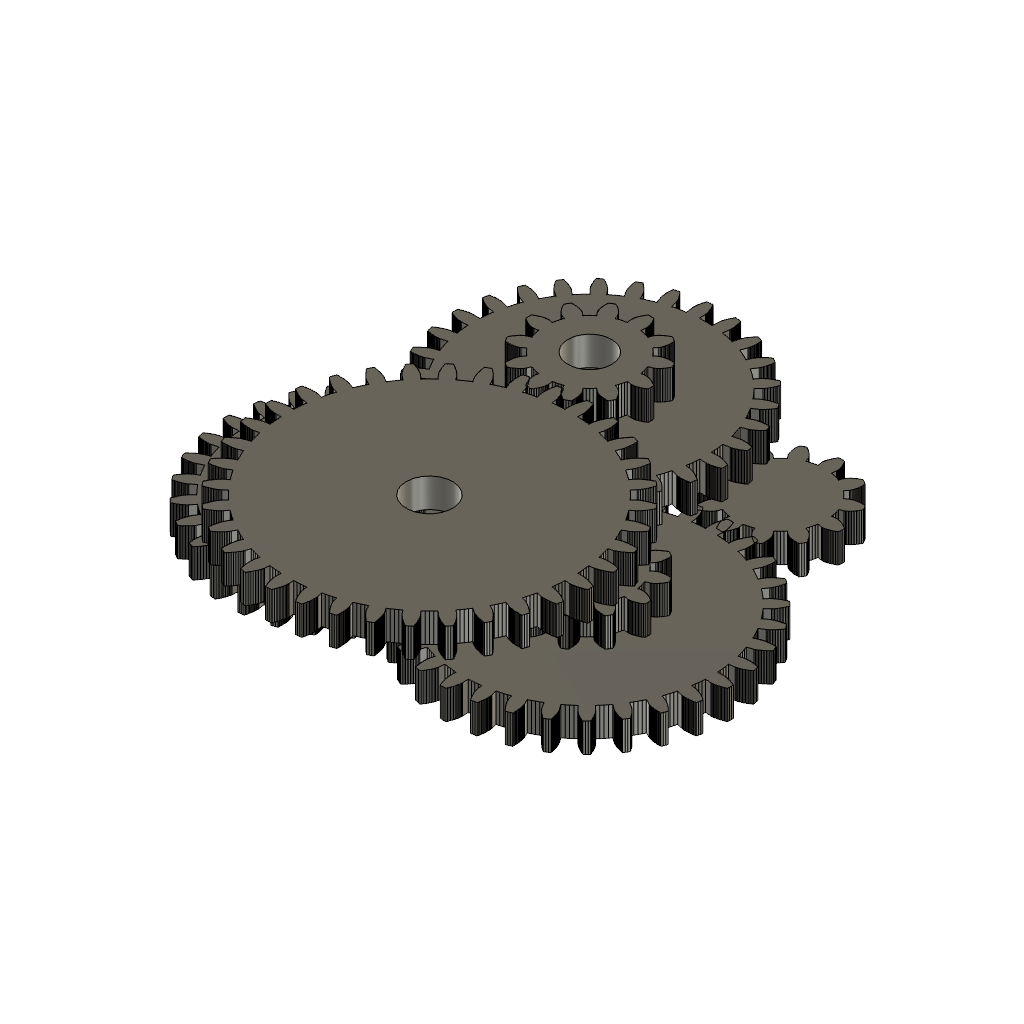
Infidex176V-IDENTIDEM.design-remix-counter-train (Autodesk Fusion 360 design; units mm, degrees)
part number: 2026-09-16-11-02-38-314
part number: 2026-09-16-11-02-48-603
part number: 2026-09-16-11-02-48-989
part number: 2026-09-16-11-02-51-230
part number: 2026-09-16-11-02-54-507
part number: 2026-09-16-11-02-59-213
Autodesk Fusion 360 part; units mm, degrees
(part 1 of 7)
ref_plane "WorkPlane1" through (0, 0, 36.8) normal (0, 0, 1) x (1, 0, 0) in component "CT sprocket pinion (tool body)"
sketch "Sketch1" plane through (0, 0, 36.8) normal (0, 0, 1) x (1, 0, 0) in component "CT sprocket pinion (tool body)"
  line L0 (76.254, -45.68) -> (76.5435, -45.7246)
  line L1 (76.5435, -45.7246) -> (76.6148, -45.7257)
  line L2 (76.6148, -45.7257) -> (76.6872, -45.7186)
  line L3 (76.6872, -45.7186) -> (76.7603, -45.7057)
  line L4 (76.7603, -45.7057) -> (76.834, -45.688)
  line L5 (76.834, -45.688) -> (76.9079, -45.6659)
  line L6 (76.9079, -45.6659) -> (76.9821, -45.6396)
  line L7 (76.9821, -45.6396) -> (77.0564, -45.6095)
  line L8 (77.0564, -45.6095) -> (77.1307, -45.5756)
  line L9 (77.1307, -45.5756) -> (77.2048, -45.538)
  line L10 (77.2048, -45.538) -> (77.2787, -45.4969)
  line L11 (77.2787, -45.4969) -> (77.3523, -45.4524)
  line L12 (77.3523, -45.4524) -> (77.4255, -45.4044)
  line L13 (77.4255, -45.4044) -> (77.4295, -45.2748)
  line L14 (77.4295, -45.2748) -> (77.4295, -45.1452)
  line L15 (77.4295, -45.1452) -> (77.4255, -45.0156)
  line L16 (77.4255, -45.0156) -> (77.3523, -44.9676)
  line L17 (77.3523, -44.9676) -> (77.2787, -44.9231)
  line L18 (77.2787, -44.9231) -> (77.2048, -44.882)
  line L19 (77.2048, -44.882) -> (77.1307, -44.8444)
  line L20 (77.1307, -44.8444) -> (77.0564, -44.8105)
  line L21 (77.0564, -44.8105) -> (76.9821, -44.7804)
  line L22 (76.9821, -44.7804) -> (76.9079, -44.7541)
  line L23 (76.9079, -44.7541) -> (76.834, -44.732)
  line L24 (76.834, -44.732) -> (76.7603, -44.7143)
  line L25 (76.7603, -44.7143) -> (76.6872, -44.7014)
  line L26 (76.6872, -44.7014) -> (76.6148, -44.6943)
  line L27 (76.6148, -44.6943) -> (76.5435, -44.6954)
  line L28 (76.5435, -44.6954) -> (76.254, -44.74)
  line L29 (76.254, -44.74) -> (76.2239, -44.5742)
  line L30 (76.2239, -44.5742) -> (76.1847, -44.4102)
  line L31 (76.1847, -44.4102) -> (76.1367, -44.2487)
  line L32 (76.1367, -44.2487) -> (76.0799, -44.09)
  line L33 (76.0799, -44.09) -> (76.3529, -43.9839)
  line L34 (76.3529, -43.9839) -> (76.4151, -43.9492)
  line L35 (76.4151, -43.9492) -> (76.4743, -43.9068)
  line L36 (76.4743, -43.9068) -> (76.5312, -43.8591)
  line L37 (76.5312, -43.8591) -> (76.5861, -43.807)
  line L38 (76.5861, -43.807) -> (76.6391, -43.7508)
  line L39 (76.6391, -43.7508) -> (76.6902, -43.691)
  line L40 (76.6902, -43.691) -> (76.7395, -43.6278)
  line L41 (76.7395, -43.6278) -> (76.7868, -43.5613)
  line L42 (76.7868, -43.5613) -> (76.8323, -43.4917)
  line L43 (76.8323, -43.4917) -> (76.8758, -43.4191)
  line L44 (76.8758, -43.4191) -> (76.9172, -43.3437)
  line L45 (76.9172, -43.3437) -> (76.9566, -43.2656)
  line L46 (76.9566, -43.2656) -> (76.8953, -43.1514)
  line L47 (76.8953, -43.1514) -> (76.8305, -43.0391)
  line L48 (76.8305, -43.0391) -> (76.7622, -42.9289)
  line L49 (76.7622, -42.9289) -> (76.6749, -42.9239)
  line L50 (76.6749, -42.9239) -> (76.5888, -42.9221)
  line L51 (76.5888, -42.9221) -> (76.5042, -42.9235)
  line L52 (76.5042, -42.9235) -> (76.4213, -42.9281)
  line L53 (76.4213, -42.9281) -> (76.34, -42.9358)
  line L54 (76.34, -42.9358) -> (76.2606, -42.9469)
  line L55 (76.2606, -42.9469) -> (76.1832, -42.9612)
  line L56 (76.1832, -42.9612) -> (76.1081, -42.9791)
  line L57 (76.1081, -42.9791) -> (76.0355, -43.0005)
  line L58 (76.0355, -43.0005) -> (75.9657, -43.026)
  line L59 (75.9657, -43.026) -> (75.8994, -43.056)
  line L60 (75.8994, -43.056) -> (75.8383, -43.0926)
  line L61 (75.8383, -43.0926) -> (75.6099, -43.2759)
  line L62 (75.6099, -43.2759) -> (75.5008, -43.1474)
  line L63 (75.5008, -43.1474) -> (75.385, -43.025)
  line L64 (75.385, -43.025) -> (75.2626, -42.9092)
  line L65 (75.2626, -42.9092) -> (75.1341, -42.8001)
  line L66 (75.1341, -42.8001) -> (75.3174, -42.5717)
  line L67 (75.3174, -42.5717) -> (75.354, -42.5106)
  line L68 (75.354, -42.5106) -> (75.384, -42.4443)
  line L69 (75.384, -42.4443) -> (75.4095, -42.3745)
  line L70 (75.4095, -42.3745) -> (75.4309, -42.3019)
  line L71 (75.4309, -42.3019) -> (75.4488, -42.2268)
  line L72 (75.4488, -42.2268) -> (75.4631, -42.1494)
  line L73 (75.4631, -42.1494) -> (75.4742, -42.07)
  line L74 (75.4742, -42.07) -> (75.4819, -41.9887)
  line L75 (75.4819, -41.9887) -> (75.4865, -41.9058)
  line L76 (75.4865, -41.9058) -> (75.4879, -41.8212)
  line L77 (75.4879, -41.8212) -> (75.4861, -41.7351)
  line L78 (75.4861, -41.7351) -> (75.4811, -41.6478)
  line L79 (75.4811, -41.6478) -> (75.3709, -41.5795)
  line L80 (75.3709, -41.5795) -> (75.2586, -41.5147)
  line L81 (75.2586, -41.5147) -> (75.1444, -41.4534)
  line L82 (75.1444, -41.4534) -> (75.0663, -41.4928)
  line L83 (75.0663, -41.4928) -> (74.9909, -41.5342)
  line L84 (74.9909, -41.5342) -> (74.9183, -41.5777)
  line L85 (74.9183, -41.5777) -> (74.8487, -41.6232)
  line L86 (74.8487, -41.6232) -> (74.7822, -41.6705)
  line L87 (74.7822, -41.6705) -> (74.719, -41.7198)
  line L88 (74.719, -41.7198) -> (74.6592, -41.7709)
  line L89 (74.6592, -41.7709) -> (74.603, -41.8239)
  line L90 (74.603, -41.8239) -> (74.5509, -41.8788)
  line L91 (74.5509, -41.8788) -> (74.5032, -41.9357)
  line L92 (74.5032, -41.9357) -> (74.4608, -41.9949)
  line L93 (74.4608, -41.9949) -> (74.4261, -42.0571)
  line L94 (74.4261, -42.0571) -> (74.32, -42.3301)
  line L95 (74.32, -42.3301) -> (74.1613, -42.2733)
  line L96 (74.1613, -42.2733) -> (73.9998, -42.2253)
  line L97 (73.9998, -42.2253) -> (73.8358, -42.1861)
  line L98 (73.8358, -42.1861) -> (73.67, -42.156)
  line L99 (73.67, -42.156) -> (73.7146, -41.8665)
  line L100 (73.7146, -41.8665) -> (73.7157, -41.7952)
  line L101 (73.7157, -41.7952) -> (73.7086, -41.7228)
  line L102 (73.7086, -41.7228) -> (73.6957, -41.6497)
  line L103 (73.6957, -41.6497) -> (73.678, -41.576)
  line L104 (73.678, -41.576) -> (73.6559, -41.5021)
  line L105 (73.6559, -41.5021) -> (73.6296, -41.4279)
  line L106 (73.6296, -41.4279) -> (73.5995, -41.3536)
  line L107 (73.5995, -41.3536) -> (73.5656, -41.2793)
  line L108 (73.5656, -41.2793) -> (73.528, -41.2052)
  line L109 (73.528, -41.2052) -> (73.4869, -41.1313)
  line L110 (73.4869, -41.1313) -> (73.4424, -41.0577)
  line L111 (73.4424, -41.0577) -> (73.3944, -40.9845)
  line L112 (73.3944, -40.9845) -> (73.2648, -40.9805)
  line L113 (73.2648, -40.9805) -> (73.1352, -40.9805)
  line L114 (73.1352, -40.9805) -> (73.0056, -40.9845)
  line L115 (73.0056, -40.9845) -> (72.9576, -41.0577)
  line L116 (72.9576, -41.0577) -> (72.9131, -41.1313)
  line L117 (72.9131, -41.1313) -> (72.872, -41.2052)
  line L118 (72.872, -41.2052) -> (72.8344, -41.2793)
  line L119 (72.8344, -41.2793) -> (72.8005, -41.3536)
  line L120 (72.8005, -41.3536) -> (72.7704, -41.4279)
  line L121 (72.7704, -41.4279) -> (72.7441, -41.5021)
  line L122 (72.7441, -41.5021) -> (72.722, -41.576)
  line L123 (72.722, -41.576) -> (72.7043, -41.6497)
  line L124 (72.7043, -41.6497) -> (72.6914, -41.7228)
  line L125 (72.6914, -41.7228) -> (72.6843, -41.7952)
  line L126 (72.6843, -41.7952) -> (72.6854, -41.8665)
  line L127 (72.6854, -41.8665) -> (72.73, -42.156)
  line L128 (72.73, -42.156) -> (72.5642, -42.1861)
  line L129 (72.5642, -42.1861) -> (72.4002, -42.2253)
  line L130 (72.4002, -42.2253) -> (72.2387, -42.2733)
  line L131 (72.2387, -42.2733) -> (72.08, -42.3301)
  line L132 (72.08, -42.3301) -> (71.9739, -42.0571)
  line L133 (71.9739, -42.0571) -> (71.9392, -41.9949)
  line L134 (71.9392, -41.9949) -> (71.8968, -41.9357)
  line L135 (71.8968, -41.9357) -> (71.8491, -41.8788)
  line L136 (71.8491, -41.8788) -> (71.797, -41.8239)
  line L137 (71.797, -41.8239) -> (71.7408, -41.7709)
  line L138 (71.7408, -41.7709) -> (71.681, -41.7198)
  line L139 (71.681, -41.7198) -> (71.6178, -41.6705)
  line L140 (71.6178, -41.6705) -> (71.5513, -41.6232)
  line L141 (71.5513, -41.6232) -> (71.4817, -41.5777)
  line L142 (71.4817, -41.5777) -> (71.4091, -41.5342)
  line L143 (71.4091, -41.5342) -> (71.3337, -41.4928)
  line L144 (71.3337, -41.4928) -> (71.2556, -41.4534)
  line L145 (71.2556, -41.4534) -> (71.1414, -41.5147)
  line L146 (71.1414, -41.5147) -> (71.0291, -41.5795)
  line L147 (71.0291, -41.5795) -> (70.9189, -41.6478)
  line L148 (70.9189, -41.6478) -> (70.9139, -41.7351)
  line L149 (70.9139, -41.7351) -> (70.9121, -41.8212)
  line L150 (70.9121, -41.8212) -> (70.9135, -41.9058)
  line L151 (70.9135, -41.9058) -> (70.9181, -41.9887)
  line L152 (70.9181, -41.9887) -> (70.9258, -42.07)
  line L153 (70.9258, -42.07) -> (70.9369, -42.1494)
  line L154 (70.9369, -42.1494) -> (70.9512, -42.2268)
  line L155 (70.9512, -42.2268) -> (70.9691, -42.3019)
  line L156 (70.9691, -42.3019) -> (70.9905, -42.3745)
  line L157 (70.9905, -42.3745) -> (71.016, -42.4443)
  line L158 (71.016, -42.4443) -> (71.046, -42.5106)
  line L159 (71.046, -42.5106) -> (71.0826, -42.5717)
  line L160 (71.0826, -42.5717) -> (71.2659, -42.8001)
  line L161 (71.2659, -42.8001) -> (71.1374, -42.9092)
  line L162 (71.1374, -42.9092) -> (71.015, -43.025)
  line L163 (71.015, -43.025) -> (70.8992, -43.1474)
  line L164 (70.8992, -43.1474) -> (70.7901, -43.2759)
  line L165 (70.7901, -43.2759) -> (70.5617, -43.0926)
  line L166 (70.5617, -43.0926) -> (70.5006, -43.056)
  line L167 (70.5006, -43.056) -> (70.4343, -43.026)
  line L168 (70.4343, -43.026) -> (70.3645, -43.0005)
  line L169 (70.3645, -43.0005) -> (70.2919, -42.9791)
  line L170 (70.2919, -42.9791) -> (70.2168, -42.9612)
  line L171 (70.2168, -42.9612) -> (70.1394, -42.9469)
  line L172 (70.1394, -42.9469) -> (70.06, -42.9358)
  line L173 (70.06, -42.9358) -> (69.9787, -42.9281)
  line L174 (69.9787, -42.9281) -> (69.8958, -42.9235)
  line L175 (69.8958, -42.9235) -> (69.8112, -42.9221)
  line L176 (69.8112, -42.9221) -> (69.7251, -42.9239)
  line L177 (69.7251, -42.9239) -> (69.6378, -42.9289)
  line L178 (69.6378, -42.9289) -> (69.5695, -43.0391)
  line L179 (69.5695, -43.0391) -> (69.5047, -43.1514)
  line L180 (69.5047, -43.1514) -> (69.4434, -43.2656)
  line L181 (69.4434, -43.2656) -> (69.4828, -43.3437)
  line L182 (69.4828, -43.3437) -> (69.5242, -43.4191)
  line L183 (69.5242, -43.4191) -> (69.5677, -43.4917)
  line L184 (69.5677, -43.4917) -> (69.6132, -43.5613)
  line L185 (69.6132, -43.5613) -> (69.6605, -43.6278)
  line L186 (69.6605, -43.6278) -> (69.7098, -43.691)
  line L187 (69.7098, -43.691) -> (69.7609, -43.7508)
  line L188 (69.7609, -43.7508) -> (69.8139, -43.807)
  line L189 (69.8139, -43.807) -> (69.8688, -43.8591)
  line L190 (69.8688, -43.8591) -> (69.9257, -43.9068)
  line L191 (69.9257, -43.9068) -> (69.9849, -43.9492)
  line L192 (69.9849, -43.9492) -> (70.0471, -43.9839)
  line L193 (70.0471, -43.9839) -> (70.3201, -44.09)
  line L194 (70.3201, -44.09) -> (70.2633, -44.2487)
  line L195 (70.2633, -44.2487) -> (70.2153, -44.4102)
  line L196 (70.2153, -44.4102) -> (70.1761, -44.5742)
  line L197 (70.1761, -44.5742) -> (70.146, -44.74)
  line L198 (70.146, -44.74) -> (69.8565, -44.6954)
  line L199 (69.8565, -44.6954) -> (69.7852, -44.6943)
  line L200 (69.7852, -44.6943) -> (69.7128, -44.7014)
  line L201 (69.7128, -44.7014) -> (69.6397, -44.7143)
  line L202 (69.6397, -44.7143) -> (69.566, -44.732)
  line L203 (69.566, -44.732) -> (69.4921, -44.7541)
  line L204 (69.4921, -44.7541) -> (69.4179, -44.7804)
  line L205 (69.4179, -44.7804) -> (69.3436, -44.8105)
  line L206 (69.3436, -44.8105) -> (69.2693, -44.8444)
  line L207 (69.2693, -44.8444) -> (69.1952, -44.882)
  line L208 (69.1952, -44.882) -> (69.1213, -44.9231)
  line L209 (69.1213, -44.9231) -> (69.0477, -44.9676)
  line L210 (69.0477, -44.9676) -> (68.9745, -45.0156)
  line L211 (68.9745, -45.0156) -> (68.9705, -45.1452)
  line L212 (68.9705, -45.1452) -> (68.9705, -45.2748)
  line L213 (68.9705, -45.2748) -> (68.9745, -45.4044)
  line L214 (68.9745, -45.4044) -> (69.0477, -45.4524)
  line L215 (69.0477, -45.4524) -> (69.1213, -45.4969)
  line L216 (69.1213, -45.4969) -> (69.1952, -45.538)
  line L217 (69.1952, -45.538) -> (69.2693, -45.5756)
  line L218 (69.2693, -45.5756) -> (69.3436, -45.6095)
  line L219 (69.3436, -45.6095) -> (69.4179, -45.6396)
  line L220 (69.4179, -45.6396) -> (69.4921, -45.6659)
  line L221 (69.4921, -45.6659) -> (69.566, -45.688)
  line L222 (69.566, -45.688) -> (69.6397, -45.7057)
  line L223 (69.6397, -45.7057) -> (69.7128, -45.7186)
  line L224 (69.7128, -45.7186) -> (69.7852, -45.7257)
  line L225 (69.7852, -45.7257) -> (69.8565, -45.7246)
  line L226 (69.8565, -45.7246) -> (70.146, -45.68)
  line L227 (70.146, -45.68) -> (70.1761, -45.8458)
  line L228 (70.1761, -45.8458) -> (70.2153, -46.0098)
  line L229 (70.2153, -46.0098) -> (70.2633, -46.1713)
  line L230 (70.2633, -46.1713) -> (70.3201, -46.33)
  line L231 (70.3201, -46.33) -> (70.0471, -46.4361)
  line L232 (70.0471, -46.4361) -> (69.9849, -46.4708)
  line L233 (69.9849, -46.4708) -> (69.9257, -46.5132)
  line L234 (69.9257, -46.5132) -> (69.8688, -46.5609)
  line L235 (69.8688, -46.5609) -> (69.8139, -46.613)
  line L236 (69.8139, -46.613) -> (69.7609, -46.6692)
  line L237 (69.7609, -46.6692) -> (69.7098, -46.729)
  line L238 (69.7098, -46.729) -> (69.6605, -46.7922)
  line L239 (69.6605, -46.7922) -> (69.6132, -46.8587)
  line L240 (69.6132, -46.8587) -> (69.5677, -46.9283)
  line L241 (69.5677, -46.9283) -> (69.5242, -47.0009)
  line L242 (69.5242, -47.0009) -> (69.4828, -47.0763)
  line L243 (69.4828, -47.0763) -> (69.4434, -47.1544)
  line L244 (69.4434, -47.1544) -> (69.5047, -47.2686)
  line L245 (69.5047, -47.2686) -> (69.5695, -47.3809)
  line L246 (69.5695, -47.3809) -> (69.6378, -47.4911)
  line L247 (69.6378, -47.4911) -> (69.7251, -47.4961)
  line L248 (69.7251, -47.4961) -> (69.8112, -47.4979)
  line L249 (69.8112, -47.4979) -> (69.8958, -47.4965)
  line L250 (69.8958, -47.4965) -> (69.9787, -47.4919)
  line L251 (69.9787, -47.4919) -> (70.06, -47.4842)
  line L252 (70.06, -47.4842) -> (70.1394, -47.4731)
  line L253 (70.1394, -47.4731) -> (70.2168, -47.4588)
  line L254 (70.2168, -47.4588) -> (70.2919, -47.4409)
  line L255 (70.2919, -47.4409) -> (70.3645, -47.4195)
  line L256 (70.3645, -47.4195) -> (70.4343, -47.394)
  line L257 (70.4343, -47.394) -> (70.5006, -47.364)
  line L258 (70.5006, -47.364) -> (70.5617, -47.3274)
  line L259 (70.5617, -47.3274) -> (70.7901, -47.1441)
  line L260 (70.7901, -47.1441) -> (70.8992, -47.2726)
  line L261 (70.8992, -47.2726) -> (71.015, -47.395)
  line L262 (71.015, -47.395) -> (71.1374, -47.5108)
  line L263 (71.1374, -47.5108) -> (71.2659, -47.6199)
  line L264 (71.2659, -47.6199) -> (71.0826, -47.8483)
  line L265 (71.0826, -47.8483) -> (71.046, -47.9094)
  line L266 (71.046, -47.9094) -> (71.016, -47.9757)
  line L267 (71.016, -47.9757) -> (70.9905, -48.0455)
  line L268 (70.9905, -48.0455) -> (70.9691, -48.1181)
  line L269 (70.9691, -48.1181) -> (70.9512, -48.1932)
  line L270 (70.9512, -48.1932) -> (70.9369, -48.2706)
  line L271 (70.9369, -48.2706) -> (70.9258, -48.35)
  line L272 (70.9258, -48.35) -> (70.9181, -48.4313)
  line L273 (70.9181, -48.4313) -> (70.9135, -48.5142)
  line L274 (70.9135, -48.5142) -> (70.9121, -48.5988)
  line L275 (70.9121, -48.5988) -> (70.9139, -48.6849)
  line L276 (70.9139, -48.6849) -> (70.9189, -48.7722)
  line L277 (70.9189, -48.7722) -> (71.0291, -48.8405)
  line L278 (71.0291, -48.8405) -> (71.1414, -48.9053)
  line L279 (71.1414, -48.9053) -> (71.2556, -48.9666)
  line L280 (71.2556, -48.9666) -> (71.3337, -48.9272)
  line L281 (71.3337, -48.9272) -> (71.4091, -48.8858)
  line L282 (71.4091, -48.8858) -> (71.4817, -48.8423)
  line L283 (71.4817, -48.8423) -> (71.5513, -48.7968)
  line L284 (71.5513, -48.7968) -> (71.6178, -48.7495)
  line L285 (71.6178, -48.7495) -> (71.681, -48.7002)
  line L286 (71.681, -48.7002) -> (71.7408, -48.6491)
  line L287 (71.7408, -48.6491) -> (71.797, -48.5961)
  line L288 (71.797, -48.5961) -> (71.8491, -48.5412)
  line L289 (71.8491, -48.5412) -> (71.8968, -48.4843)
  line L290 (71.8968, -48.4843) -> (71.9392, -48.4251)
  line L291 (71.9392, -48.4251) -> (71.9739, -48.3629)
  line L292 (71.9739, -48.3629) -> (72.08, -48.0899)
  line L293 (72.08, -48.0899) -> (72.2387, -48.1467)
  line L294 (72.2387, -48.1467) -> (72.4002, -48.1947)
  line L295 (72.4002, -48.1947) -> (72.5642, -48.2339)
  line L296 (72.5642, -48.2339) -> (72.73, -48.264)
  line L297 (72.73, -48.264) -> (72.6854, -48.5535)
  line L298 (72.6854, -48.5535) -> (72.6843, -48.6248)
  line L299 (72.6843, -48.6248) -> (72.6914, -48.6972)
  line L300 (72.6914, -48.6972) -> (72.7043, -48.7703)
  line L301 (72.7043, -48.7703) -> (72.722, -48.844)
  line L302 (72.722, -48.844) -> (72.7441, -48.9179)
  line L303 (72.7441, -48.9179) -> (72.7704, -48.9921)
  line L304 (72.7704, -48.9921) -> (72.8005, -49.0664)
  line L305 (72.8005, -49.0664) -> (72.8344, -49.1407)
  line L306 (72.8344, -49.1407) -> (72.872, -49.2148)
  line L307 (72.872, -49.2148) -> (72.9131, -49.2887)
  line L308 (72.9131, -49.2887) -> (72.9576, -49.3623)
  line L309 (72.9576, -49.3623) -> (73.0056, -49.4355)
  line L310 (73.0056, -49.4355) -> (73.1352, -49.4395)
  line L311 (73.1352, -49.4395) -> (73.2648, -49.4395)
  line L312 (73.2648, -49.4395) -> (73.3944, -49.4355)
  line L313 (73.3944, -49.4355) -> (73.4424, -49.3623)
  line L314 (73.4424, -49.3623) -> (73.4869, -49.2887)
  line L315 (73.4869, -49.2887) -> (73.528, -49.2148)
  line L316 (73.528, -49.2148) -> (73.5656, -49.1407)
  line L317 (73.5656, -49.1407) -> (73.5995, -49.0664)
  line L318 (73.5995, -49.0664) -> (73.6296, -48.9921)
  line L319 (73.6296, -48.9921) -> (73.6559, -48.9179)
  line L320 (73.6559, -48.9179) -> (73.678, -48.844)
  line L321 (73.678, -48.844) -> (73.6957, -48.7703)
  line L322 (73.6957, -48.7703) -> (73.7086, -48.6972)
  line L323 (73.7086, -48.6972) -> (73.7157, -48.6248)
  line L324 (73.7157, -48.6248) -> (73.7146, -48.5535)
  line L325 (73.7146, -48.5535) -> (73.67, -48.264)
  line L326 (73.67, -48.264) -> (73.8358, -48.2339)
  line L327 (73.8358, -48.2339) -> (73.9998, -48.1947)
  line L328 (73.9998, -48.1947) -> (74.1613, -48.1467)
  line L329 (74.1613, -48.1467) -> (74.32, -48.0899)
  line L330 (74.32, -48.0899) -> (74.4261, -48.3629)
  line L331 (74.4261, -48.3629) -> (74.4608, -48.4251)
  line L332 (74.4608, -48.4251) -> (74.5032, -48.4843)
  line L333 (74.5032, -48.4843) -> (74.5509, -48.5412)
  line L334 (74.5509, -48.5412) -> (74.603, -48.5961)
  line L335 (74.603, -48.5961) -> (74.6592, -48.6491)
  line L336 (74.6592, -48.6491) -> (74.719, -48.7002)
  line L337 (74.719, -48.7002) -> (74.7822, -48.7495)
  line L338 (74.7822, -48.7495) -> (74.8487, -48.7968)
  line L339 (74.8487, -48.7968) -> (74.9183, -48.8423)
  line L340 (74.9183, -48.8423) -> (74.9909, -48.8858)
  line L341 (74.9909, -48.8858) -> (75.0663, -48.9272)
  line L342 (75.0663, -48.9272) -> (75.1444, -48.9666)
  line L343 (75.1444, -48.9666) -> (75.2586, -48.9053)
  line L344 (75.2586, -48.9053) -> (75.3709, -48.8405)
  line L345 (75.3709, -48.8405) -> (75.4811, -48.7722)
  line L346 (75.4811, -48.7722) -> (75.4861, -48.6849)
  line L347 (75.4861, -48.6849) -> (75.4879, -48.5988)
  line L348 (75.4879, -48.5988) -> (75.4865, -48.5142)
  line L349 (75.4865, -48.5142) -> (75.4819, -48.4313)
  line L350 (75.4819, -48.4313) -> (75.4742, -48.35)
  line L351 (75.4742, -48.35) -> (75.4631, -48.2706)
  line L352 (75.4631, -48.2706) -> (75.4488, -48.1932)
  line L353 (75.4488, -48.1932) -> (75.4309, -48.1181)
  line L354 (75.4309, -48.1181) -> (75.4095, -48.0455)
  line L355 (75.4095, -48.0455) -> (75.384, -47.9757)
  line L356 (75.384, -47.9757) -> (75.354, -47.9094)
  line L357 (75.354, -47.9094) -> (75.3174, -47.8483)
  line L358 (75.3174, -47.8483) -> (75.1341, -47.6199)
  line L359 (75.1341, -47.6199) -> (75.2626, -47.5108)
  line L360 (75.2626, -47.5108) -> (75.385, -47.395)
  line L361 (75.385, -47.395) -> (75.5008, -47.2726)
  line L362 (75.5008, -47.2726) -> (75.6099, -47.1441)
  line L363 (75.6099, -47.1441) -> (75.8383, -47.3274)
  line L364 (75.8383, -47.3274) -> (75.8994, -47.364)
  line L365 (75.8994, -47.364) -> (75.9657, -47.394)
  line L366 (75.9657, -47.394) -> (76.0355, -47.4195)
  line L367 (76.0355, -47.4195) -> (76.1081, -47.4409)
  line L368 (76.1081, -47.4409) -> (76.1832, -47.4588)
  line L369 (76.1832, -47.4588) -> (76.2606, -47.4731)
  line L370 (76.2606, -47.4731) -> (76.34, -47.4842)
  line L371 (76.34, -47.4842) -> (76.4213, -47.4919)
  line L372 (76.4213, -47.4919) -> (76.5042, -47.4965)
  line L373 (76.5042, -47.4965) -> (76.5888, -47.4979)
  line L374 (76.5888, -47.4979) -> (76.6749, -47.4961)
  line L375 (76.6749, -47.4961) -> (76.7622, -47.4911)
  line L376 (76.7622, -47.4911) -> (76.8305, -47.3809)
  line L377 (76.8305, -47.3809) -> (76.8953, -47.2686)
  line L378 (76.8953, -47.2686) -> (76.9566, -47.1544)
  line L379 (76.9566, -47.1544) -> (76.9172, -47.0763)
  line L380 (76.9172, -47.0763) -> (76.8758, -47.0009)
  line L381 (76.8758, -47.0009) -> (76.8323, -46.9283)
  line L382 (76.8323, -46.9283) -> (76.7868, -46.8587)
  line L383 (76.7868, -46.8587) -> (76.7395, -46.7922)
  line L384 (76.7395, -46.7922) -> (76.6902, -46.729)
  line L385 (76.6902, -46.729) -> (76.6391, -46.6692)
  line L386 (76.6391, -46.6692) -> (76.5861, -46.613)
  line L387 (76.5861, -46.613) -> (76.5312, -46.5609)
  line L388 (76.5312, -46.5609) -> (76.4743, -46.5132)
  line L389 (76.4743, -46.5132) -> (76.4151, -46.4708)
  line L390 (76.4151, -46.4708) -> (76.3529, -46.4361)
  line L391 (76.3529, -46.4361) -> (76.0799, -46.33)
  line L392 (76.0799, -46.33) -> (76.1367, -46.1713)
  line L393 (76.1367, -46.1713) -> (76.1847, -46.0098)
  line L394 (76.1847, -46.0098) -> (76.2239, -45.8458)
  line L395 (76.2239, -45.8458) -> (76.254, -45.68)
extrude "Extrude1" add sketch "Sketch1" along normal blind 2 makes body 1 in component "CT sprocket pinion (tool body)"
ref_plane "WorkPlane1" through (0, 0, 36.8) normal (0, 0, 1) x (1, 0, 0) in component "CT idler 1"
sketch "Sketch1 (2)" plane through (0, 0, 36.8) normal (0, 0, 1) x (1, 0, 0) in component "CT idler 1"
  line L0 (81.6294, -58.8253) -> (82.04, -58.8452)
  line L1 (82.04, -58.8452) -> (82.1151, -58.8424)
  line L2 (82.1151, -58.8424) -> (82.1905, -58.8341)
  line L3 (82.1905, -58.8341) -> (82.2661, -58.8222)
  line L4 (82.2661, -58.8222) -> (82.3417, -58.8073)
  line L5 (82.3417, -58.8073) -> (82.4174, -58.7898)
  line L6 (82.4174, -58.7898) -> (82.4932, -58.7699)
  line L7 (82.4932, -58.7699) -> (82.5689, -58.7477)
  line L8 (82.5689, -58.7477) -> (82.6447, -58.7234)
  line L9 (82.6447, -58.7234) -> (82.7205, -58.6971)
  line L10 (82.7205, -58.6971) -> (82.7962, -58.6689)
  line L11 (82.7962, -58.6689) -> (82.8719, -58.6389)
  line L12 (82.8719, -58.6389) -> (82.9475, -58.607)
  line L13 (82.9475, -58.607) -> (82.9493, -58.4749)
  line L14 (82.9493, -58.4749) -> (82.9493, -58.3429)
  line L15 (82.9493, -58.3429) -> (82.9475, -58.2108)
  line L16 (82.9475, -58.2108) -> (82.8719, -58.1789)
  line L17 (82.8719, -58.1789) -> (82.7962, -58.1489)
  line L18 (82.7962, -58.1489) -> (82.7205, -58.1207)
  line L19 (82.7205, -58.1207) -> (82.6447, -58.0944)
  line L20 (82.6447, -58.0944) -> (82.5689, -58.0701)
  line L21 (82.5689, -58.0701) -> (82.4932, -58.0479)
  line L22 (82.4932, -58.0479) -> (82.4174, -58.028)
  line L23 (82.4174, -58.028) -> (82.3417, -58.0105)
  line L24 (82.3417, -58.0105) -> (82.2661, -57.9956)
  line L25 (82.2661, -57.9956) -> (82.1905, -57.9837)
  line L26 (82.1905, -57.9837) -> (82.1151, -57.9754)
  line L27 (82.1151, -57.9754) -> (82.04, -57.9726)
  line L28 (82.04, -57.9726) -> (81.6294, -57.9925)
  line L29 (81.6294, -57.9925) -> (81.6164, -57.7785)
  line L30 (81.6164, -57.7785) -> (81.5981, -57.565)
  line L31 (81.5981, -57.565) -> (81.5744, -57.3519)
  line L32 (81.5744, -57.3519) -> (81.5454, -57.1395)
  line L33 (81.5454, -57.1395) -> (81.952, -57.0789)
  line L34 (81.952, -57.0789) -> (82.0251, -57.0615)
  line L35 (82.0251, -57.0615) -> (82.0975, -57.0387)
  line L36 (82.0975, -57.0387) -> (82.1692, -57.0123)
  line L37 (82.1692, -57.0123) -> (82.2405, -56.9829)
  line L38 (82.2405, -56.9829) -> (82.3113, -56.951)
  line L39 (82.3113, -56.951) -> (82.3817, -56.9167)
  line L40 (82.3817, -56.9167) -> (82.4517, -56.8801)
  line L41 (82.4517, -56.8801) -> (82.5213, -56.8416)
  line L42 (82.5213, -56.8416) -> (82.5905, -56.801)
  line L43 (82.5905, -56.801) -> (82.6593, -56.7585)
  line L44 (82.6593, -56.7585) -> (82.7277, -56.7143)
  line L45 (82.7277, -56.7143) -> (82.7956, -56.6683)
  line L46 (82.7956, -56.6683) -> (82.7716, -56.5384)
  line L47 (82.7716, -56.5384) -> (82.7458, -56.4089)
  line L48 (82.7458, -56.4089) -> (82.7183, -56.2797)
  line L49 (82.7183, -56.2797) -> (82.6379, -56.2632)
  line L50 (82.6379, -56.2632) -> (82.5578, -56.2485)
  line L51 (82.5578, -56.2485) -> (82.4781, -56.2356)
  line L52 (82.4781, -56.2356) -> (82.3986, -56.2246)
  line L53 (82.3986, -56.2246) -> (82.3195, -56.2156)
  line L54 (82.3195, -56.2156) -> (82.2409, -56.2086)
  line L55 (82.2409, -56.2086) -> (82.1627, -56.2038)
  line L56 (82.1627, -56.2038) -> (82.085, -56.2014)
  line L57 (82.085, -56.2014) -> (82.008, -56.2016)
  line L58 (82.008, -56.2016) -> (81.9316, -56.2047)
  line L59 (81.9316, -56.2047) -> (81.856, -56.2113)
  line L60 (81.856, -56.2113) -> (81.7818, -56.2231)
  line L61 (81.7818, -56.2231) -> (81.383, -56.3227)
  line L62 (81.383, -56.3227) -> (81.3284, -56.1154)
  line L63 (81.3284, -56.1154) -> (81.2688, -55.9095)
  line L64 (81.2688, -55.9095) -> (81.204, -55.7052)
  line L65 (81.204, -55.7052) -> (81.1342, -55.5026)
  line L66 (81.1342, -55.5026) -> (81.5211, -55.3638)
  line L67 (81.5211, -55.3638) -> (81.5894, -55.3324)
  line L68 (81.5894, -55.3324) -> (81.6559, -55.2959)
  line L69 (81.6559, -55.2959) -> (81.7211, -55.2561)
  line L70 (81.7211, -55.2561) -> (81.7853, -55.2134)
  line L71 (81.7853, -55.2134) -> (81.8486, -55.1682)
  line L72 (81.8486, -55.1682) -> (81.9109, -55.1208)
  line L73 (81.9109, -55.1208) -> (81.9725, -55.0713)
  line L74 (81.9725, -55.0713) -> (82.0332, -55.0199)
  line L75 (82.0332, -55.0199) -> (82.0931, -54.9666)
  line L76 (82.0931, -54.9666) -> (82.1523, -54.9116)
  line L77 (82.1523, -54.9116) -> (82.2107, -54.8548)
  line L78 (82.2107, -54.8548) -> (82.2684, -54.7964)
  line L79 (82.2684, -54.7964) -> (82.2195, -54.6738)
  line L80 (82.2195, -54.6738) -> (82.1689, -54.5518)
  line L81 (82.1689, -54.5518) -> (82.1168, -54.4304)
  line L82 (82.1168, -54.4304) -> (82.0347, -54.4299)
  line L83 (82.0347, -54.4299) -> (81.9533, -54.4311)
  line L84 (81.9533, -54.4311) -> (81.8725, -54.434)
  line L85 (81.8725, -54.434) -> (81.7924, -54.4387)
  line L86 (81.7924, -54.4387) -> (81.7131, -54.4453)
  line L87 (81.7131, -54.4453) -> (81.6347, -54.4538)
  line L88 (81.6347, -54.4538) -> (81.557, -54.4644)
  line L89 (81.557, -54.4644) -> (81.4804, -54.4772)
  line L90 (81.4804, -54.4772) -> (81.4048, -54.4924)
  line L91 (81.4048, -54.4924) -> (81.3305, -54.5103)
  line L92 (81.3305, -54.5103) -> (81.2577, -54.5315)
  line L93 (81.2577, -54.5315) -> (81.1872, -54.5577)
  line L94 (81.1872, -54.5577) -> (80.8155, -54.7331)
  line L95 (80.8155, -54.7331) -> (80.7215, -54.5405)
  line L96 (80.7215, -54.5405) -> (80.6229, -54.3502)
  line L97 (80.6229, -54.3502) -> (80.5195, -54.1624)
  line L98 (80.5195, -54.1624) -> (80.4114, -53.9773)
  line L99 (80.4114, -53.9773) -> (80.7639, -53.7657)
  line L100 (80.7639, -53.7657) -> (80.8248, -53.7216)
  line L101 (80.8248, -53.7216) -> (80.8828, -53.6728)
  line L102 (80.8828, -53.6728) -> (80.939, -53.621)
  line L103 (80.939, -53.621) -> (80.9937, -53.5666)
  line L104 (80.9937, -53.5666) -> (81.0469, -53.51)
  line L105 (81.0469, -53.51) -> (81.0988, -53.4513)
  line L106 (81.0988, -53.4513) -> (81.1495, -53.3908)
  line L107 (81.1495, -53.3908) -> (81.199, -53.3285)
  line L108 (81.199, -53.3285) -> (81.2474, -53.2646)
  line L109 (81.2474, -53.2646) -> (81.2947, -53.199)
  line L110 (81.2947, -53.199) -> (81.3409, -53.132)
  line L111 (81.3409, -53.132) -> (81.3861, -53.0634)
  line L112 (81.3861, -53.0634) -> (81.3142, -52.9527)
  line L113 (81.3142, -52.9527) -> (81.2408, -52.8429)
  line L114 (81.2408, -52.8429) -> (81.166, -52.734)
  line L115 (81.166, -52.734) -> (81.0854, -52.7495)
  line L116 (81.0854, -52.7495) -> (81.0058, -52.7666)
  line L117 (81.0058, -52.7666) -> (80.9271, -52.7852)
  line L118 (80.9271, -52.7852) -> (80.8495, -52.8055)
  line L119 (80.8495, -52.8055) -> (80.773, -52.8274)
  line L120 (80.773, -52.8274) -> (80.6977, -52.851)
  line L121 (80.6977, -52.851) -> (80.6237, -52.8766)
  line L122 (80.6237, -52.8766) -> (80.551, -52.9041)
  line L123 (80.551, -52.9041) -> (80.4798, -52.9337)
  line L124 (80.4798, -52.9337) -> (80.4104, -52.9658)
  line L125 (80.4104, -52.9658) -> (80.3431, -53.0008)
  line L126 (80.3431, -53.0008) -> (80.2791, -53.0402)
  line L127 (80.2791, -53.0402) -> (79.9488, -53.2848)
  line L128 (79.9488, -53.2848) -> (79.8191, -53.1141)
  line L129 (79.8191, -53.1141) -> (79.6851, -52.9468)
  line L130 (79.6851, -52.9468) -> (79.5471, -52.7828)
  line L131 (79.5471, -52.7828) -> (79.405, -52.6223)
  line L132 (79.405, -52.6223) -> (79.7094, -52.346)
  line L133 (79.7094, -52.346) -> (79.7605, -52.2909)
  line L134 (79.7605, -52.2909) -> (79.808, -52.2317)
  line L135 (79.808, -52.2317) -> (79.853, -52.1699)
  line L136 (79.853, -52.1699) -> (79.8959, -52.1059)
  line L137 (79.8959, -52.1059) -> (79.9371, -52.04)
  line L138 (79.9371, -52.04) -> (79.9766, -51.9723)
  line L139 (79.9766, -51.9723) -> (80.0145, -51.9031)
  line L140 (80.0145, -51.9031) -> (80.0509, -51.8323)
  line L141 (80.0509, -51.8323) -> (80.0859, -51.7602)
  line L142 (80.0859, -51.7602) -> (80.1195, -51.6867)
  line L143 (80.1195, -51.6867) -> (80.1518, -51.6119)
  line L144 (80.1518, -51.6119) -> (80.1827, -51.5359)
  line L145 (80.1827, -51.5359) -> (80.0906, -51.4412)
  line L146 (80.0906, -51.4412) -> (79.9972, -51.3479)
  line L147 (79.9972, -51.3479) -> (79.9026, -51.2557)
  line L148 (79.9026, -51.2557) -> (79.8265, -51.2867)
  line L149 (79.8265, -51.2867) -> (79.7518, -51.3189)
  line L150 (79.7518, -51.3189) -> (79.6783, -51.3525)
  line L151 (79.6783, -51.3525) -> (79.6061, -51.3875)
  line L152 (79.6061, -51.3875) -> (79.5353, -51.4239)
  line L153 (79.5353, -51.4239) -> (79.4661, -51.4619)
  line L154 (79.4661, -51.4619) -> (79.3984, -51.5013)
  line L155 (79.3984, -51.5013) -> (79.3325, -51.5425)
  line L156 (79.3325, -51.5425) -> (79.2685, -51.5854)
  line L157 (79.2685, -51.5854) -> (79.2067, -51.6304)
  line L158 (79.2067, -51.6304) -> (79.1475, -51.6779)
  line L159 (79.1475, -51.6779) -> (79.0924, -51.729)
  line L160 (79.0924, -51.729) -> (78.8161, -52.0334)
  line L161 (78.8161, -52.0334) -> (78.6556, -51.8913)
  line L162 (78.6556, -51.8913) -> (78.4916, -51.7533)
  line L163 (78.4916, -51.7533) -> (78.3243, -51.6194)
  line L164 (78.3243, -51.6194) -> (78.1536, -51.4897)
  line L165 (78.1536, -51.4897) -> (78.3982, -51.1593)
  line L166 (78.3982, -51.1593) -> (78.4376, -51.0953)
  line L167 (78.4376, -51.0953) -> (78.4726, -51.028)
  line L168 (78.4726, -51.028) -> (78.5047, -50.9586)
  line L169 (78.5047, -50.9586) -> (78.5344, -50.8874)
  line L170 (78.5344, -50.8874) -> (78.5619, -50.8148)
  line L171 (78.5619, -50.8148) -> (78.5874, -50.7407)
  line L172 (78.5874, -50.7407) -> (78.611, -50.6654)
  line L173 (78.611, -50.6654) -> (78.633, -50.5889)
  line L174 (78.633, -50.5889) -> (78.6532, -50.5113)
  line L175 (78.6532, -50.5113) -> (78.6718, -50.4326)
  line L176 (78.6718, -50.4326) -> (78.6889, -50.353)
  line L177 (78.6889, -50.353) -> (78.7044, -50.2724)
  line L178 (78.7044, -50.2724) -> (78.5956, -50.1976)
  line L179 (78.5956, -50.1976) -> (78.4858, -50.1242)
  line L180 (78.4858, -50.1242) -> (78.375, -50.0523)
  line L181 (78.375, -50.0523) -> (78.3065, -50.0975)
  line L182 (78.3065, -50.0975) -> (78.2394, -50.1437)
  line L183 (78.2394, -50.1437) -> (78.1739, -50.191)
  line L184 (78.1739, -50.191) -> (78.1099, -50.2394)
  line L185 (78.1099, -50.2394) -> (78.0476, -50.2889)
  line L186 (78.0476, -50.2889) -> (77.9871, -50.3396)
  line L187 (77.9871, -50.3396) -> (77.9285, -50.3915)
  line L188 (77.9285, -50.3915) -> (77.8718, -50.4448)
  line L189 (77.8718, -50.4448) -> (77.8174, -50.4994)
  line L190 (77.8174, -50.4994) -> (77.7656, -50.5556)
  line L191 (77.7656, -50.5556) -> (77.7168, -50.6137)
  line L192 (77.7168, -50.6137) -> (77.6727, -50.6746)
  line L193 (77.6727, -50.6746) -> (77.4612, -51.027)
  line L194 (77.4612, -51.027) -> (77.276, -50.9189)
  line L195 (77.276, -50.9189) -> (77.0882, -50.8156)
  line L196 (77.0882, -50.8156) -> (76.898, -50.7169)
  line L197 (76.898, -50.7169) -> (76.7053, -50.623)
  line L198 (76.7053, -50.623) -> (76.8808, -50.2512)
  line L199 (76.8808, -50.2512) -> (76.9069, -50.1807)
  line L200 (76.9069, -50.1807) -> (76.9281, -50.1079)
  line L201 (76.9281, -50.1079) -> (76.946, -50.0336)
  line L202 (76.946, -50.0336) -> (76.9612, -49.958)
  line L203 (76.9612, -49.958) -> (76.974, -49.8814)
  line L204 (76.974, -49.8814) -> (76.9846, -49.8038)
  line L205 (76.9846, -49.8038) -> (76.9931, -49.7253)
  line L206 (76.9931, -49.7253) -> (76.9997, -49.646)
  line L207 (76.9997, -49.646) -> (77.0044, -49.5659)
  line L208 (77.0044, -49.5659) -> (77.0073, -49.4851)
  line L209 (77.0073, -49.4851) -> (77.0085, -49.4037)
  line L210 (77.0085, -49.4037) -> (77.008, -49.3216)
  line L211 (77.008, -49.3216) -> (76.8867, -49.2695)
  line L212 (76.8867, -49.2695) -> (76.7647, -49.2189)
  line L213 (76.7647, -49.2189) -> (76.642, -49.17)
  line L214 (76.642, -49.17) -> (76.5836, -49.2277)
  line L215 (76.5836, -49.2277) -> (76.5268, -49.2861)
  line L216 (76.5268, -49.2861) -> (76.4718, -49.3453)
  line L217 (76.4718, -49.3453) -> (76.4185, -49.4052)
  line L218 (76.4185, -49.4052) -> (76.3671, -49.466)
  line L219 (76.3671, -49.466) -> (76.3176, -49.5275)
  line L220 (76.3176, -49.5275) -> (76.2702, -49.5899)
  line L221 (76.2702, -49.5899) -> (76.2251, -49.6531)
  line L222 (76.2251, -49.6531) -> (76.1824, -49.7173)
  line L223 (76.1824, -49.7173) -> (76.1425, -49.7825)
  line L224 (76.1425, -49.7825) -> (76.106, -49.849)
  line L225 (76.106, -49.849) -> (76.0746, -49.9173)
  line L226 (76.0746, -49.9173) -> (75.9359, -50.3043)
  line L227 (75.9359, -50.3043) -> (75.7332, -50.2344)
  line L228 (75.7332, -50.2344) -> (75.5289, -50.1696)
  line L229 (75.5289, -50.1696) -> (75.323, -50.11)
  line L230 (75.323, -50.11) -> (75.1157, -50.0555)
  line L231 (75.1157, -50.0555) -> (75.2153, -49.6567)
  line L232 (75.2153, -49.6567) -> (75.2272, -49.5824)
  line L233 (75.2272, -49.5824) -> (75.2338, -49.5069)
  line L234 (75.2338, -49.5069) -> (75.2368, -49.4305)
  line L235 (75.2368, -49.4305) -> (75.237, -49.3534)
  line L236 (75.237, -49.3534) -> (75.2346, -49.2757)
  line L237 (75.2346, -49.2757) -> (75.2298, -49.1975)
  line L238 (75.2298, -49.1975) -> (75.2229, -49.1189)
  line L239 (75.2229, -49.1189) -> (75.2138, -49.0398)
  line L240 (75.2138, -49.0398) -> (75.2028, -48.9604)
  line L241 (75.2028, -48.9604) -> (75.19, -48.8806)
  line L242 (75.19, -48.8806) -> (75.1752, -48.8005)
  line L243 (75.1752, -48.8005) -> (75.1587, -48.7201)
  line L244 (75.1587, -48.7201) -> (75.0295, -48.6926)
  line L245 (75.0295, -48.6926) -> (74.9, -48.6668)
  line L246 (74.9, -48.6668) -> (74.7702, -48.6428)
  line L247 (74.7702, -48.6428) -> (74.7241, -48.7108)
  line L248 (74.7241, -48.7108) -> (74.6799, -48.7791)
  line L249 (74.6799, -48.7791) -> (74.6374, -48.8479)
  line L250 (74.6374, -48.8479) -> (74.5969, -48.9171)
  line L251 (74.5969, -48.9171) -> (74.5583, -48.9867)
  line L252 (74.5583, -48.9867) -> (74.5218, -49.0567)
  line L253 (74.5218, -49.0567) -> (74.4874, -49.1271)
  line L254 (74.4874, -49.1271) -> (74.4555, -49.1979)
  line L255 (74.4555, -49.1979) -> (74.4261, -49.2692)
  line L256 (74.4261, -49.2692) -> (74.3997, -49.341)
  line L257 (74.3997, -49.341) -> (74.3769, -49.4133)
  line L258 (74.3769, -49.4133) -> (74.3595, -49.4864)
  line L259 (74.3595, -49.4864) -> (74.2989, -49.893)
  line L260 (74.2989, -49.893) -> (74.0865, -49.864)
  line L261 (74.0865, -49.864) -> (73.8734, -49.8404)
  line L262 (73.8734, -49.8404) -> (73.6599, -49.822)
  line L263 (73.6599, -49.822) -> (73.4459, -49.809)
  line L264 (73.4459, -49.809) -> (73.4658, -49.3984)
  line L265 (73.4658, -49.3984) -> (73.463, -49.3233)
  line L266 (73.463, -49.3233) -> (73.4547, -49.2479)
  line L267 (73.4547, -49.2479) -> (73.4428, -49.1724)
  line L268 (73.4428, -49.1724) -> (73.4279, -49.0967)
  line L269 (73.4279, -49.0967) -> (73.4104, -49.021)
  line L270 (73.4104, -49.021) -> (73.3905, -48.9453)
  line L271 (73.3905, -48.9453) -> (73.3683, -48.8695)
  line L272 (73.3683, -48.8695) -> (73.3441, -48.7937)
  line L273 (73.3441, -48.7937) -> (73.3178, -48.7179)
  line L274 (73.3178, -48.7179) -> (73.2896, -48.6422)
  line L275 (73.2896, -48.6422) -> (73.2595, -48.5665)
  line L276 (73.2595, -48.5665) -> (73.2276, -48.4909)
  line L277 (73.2276, -48.4909) -> (73.0956, -48.4891)
  line L278 (73.0956, -48.4891) -> (72.9635, -48.4891)
  line L279 (72.9635, -48.4891) -> (72.8314, -48.4909)
  line L280 (72.8314, -48.4909) -> (72.7996, -48.5665)
  line L281 (72.7996, -48.5665) -> (72.7695, -48.6422)
  line L282 (72.7695, -48.6422) -> (72.7413, -48.7179)
  line L283 (72.7413, -48.7179) -> (72.715, -48.7937)
  line L284 (72.715, -48.7937) -> (72.6907, -48.8695)
  line L285 (72.6907, -48.8695) -> (72.6686, -48.9453)
  line L286 (72.6686, -48.9453) -> (72.6486, -49.021)
  line L287 (72.6486, -49.021) -> (72.6311, -49.0967)
  line L288 (72.6311, -49.0967) -> (72.6162, -49.1724)
  line L289 (72.6162, -49.1724) -> (72.6043, -49.2479)
  line L290 (72.6043, -49.2479) -> (72.5961, -49.3233)
  line L291 (72.5961, -49.3233) -> (72.5932, -49.3984)
  line L292 (72.5932, -49.3984) -> (72.6131, -49.809)
  line L293 (72.6131, -49.809) -> (72.3992, -49.822)
  line L294 (72.3992, -49.822) -> (72.1856, -49.8404)
  line L295 (72.1856, -49.8404) -> (71.9726, -49.864)
  line L296 (71.9726, -49.864) -> (71.7602, -49.893)
  line L297 (71.7602, -49.893) -> (71.6996, -49.4864)
  line L298 (71.6996, -49.4864) -> (71.6821, -49.4133)
  line L299 (71.6821, -49.4133) -> (71.6593, -49.341)
  line L300 (71.6593, -49.341) -> (71.6329, -49.2692)
  line L301 (71.6329, -49.2692) -> (71.6036, -49.1979)
  line L302 (71.6036, -49.1979) -> (71.5716, -49.1271)
  line L303 (71.5716, -49.1271) -> (71.5373, -49.0567)
  line L304 (71.5373, -49.0567) -> (71.5008, -48.9867)
  line L305 (71.5008, -48.9867) -> (71.4622, -48.9171)
  line L306 (71.4622, -48.9171) -> (71.4216, -48.8479)
  line L307 (71.4216, -48.8479) -> (71.3792, -48.7791)
  line L308 (71.3792, -48.7791) -> (71.3349, -48.7108)
  line L309 (71.3349, -48.7108) -> (71.2889, -48.6428)
  line L310 (71.2889, -48.6428) -> (71.159, -48.6668)
  line L311 (71.159, -48.6668) -> (71.0295, -48.6926)
  line L312 (71.0295, -48.6926) -> (70.9003, -48.7201)
  line L313 (70.9003, -48.7201) -> (70.8838, -48.8005)
  line L314 (70.8838, -48.8005) -> (70.8691, -48.8806)
  line L315 (70.8691, -48.8806) -> (70.8562, -48.9604)
  line L316 (70.8562, -48.9604) -> (70.8452, -49.0398)
  line L317 (70.8452, -49.0398) -> (70.8362, -49.1189)
  line L318 (70.8362, -49.1189) -> (70.8292, -49.1975)
  line L319 (70.8292, -49.1975) -> (70.8245, -49.2757)
  line L320 (70.8245, -49.2757) -> (70.822, -49.3534)
  line L321 (70.822, -49.3534) -> (70.8222, -49.4305)
  line L322 (70.8222, -49.4305) -> (70.8253, -49.5069)
  line L323 (70.8253, -49.5069) -> (70.8319, -49.5824)
  line L324 (70.8319, -49.5824) -> (70.8438, -49.6567)
  line L325 (70.8438, -49.6567) -> (70.9434, -50.0555)
  line L326 (70.9434, -50.0555) -> (70.7361, -50.11)
  line L327 (70.7361, -50.11) -> (70.5302, -50.1696)
  line L328 (70.5302, -50.1696) -> (70.3258, -50.2344)
  line L329 (70.3258, -50.2344) -> (70.1232, -50.3043)
  line L330 (70.1232, -50.3043) -> (69.9844, -49.9173)
  line L331 (69.9844, -49.9173) -> (69.9531, -49.849)
  line L332 (69.9531, -49.849) -> (69.9166, -49.7825)
  line L333 (69.9166, -49.7825) -> (69.8767, -49.7173)
  line L334 (69.8767, -49.7173) -> (69.834, -49.6531)
  line L335 (69.834, -49.6531) -> (69.7888, -49.5899)
  line L336 (69.7888, -49.5899) -> (69.7414, -49.5275)
  line L337 (69.7414, -49.5275) -> (69.692, -49.466)
  line L338 (69.692, -49.466) -> (69.6405, -49.4052)
  line L339 (69.6405, -49.4052) -> (69.5873, -49.3453)
  line L340 (69.5873, -49.3453) -> (69.5322, -49.2861)
  line L341 (69.5322, -49.2861) -> (69.4755, -49.2277)
  line L342 (69.4755, -49.2277) -> (69.4171, -49.17)
  line L343 (69.4171, -49.17) -> (69.2944, -49.2189)
  line L344 (69.2944, -49.2189) -> (69.1724, -49.2695)
  line L345 (69.1724, -49.2695) -> (69.0511, -49.3216)
  line L346 (69.0511, -49.3216) -> (69.0505, -49.4037)
  line L347 (69.0505, -49.4037) -> (69.0517, -49.4851)
  line L348 (69.0517, -49.4851) -> (69.0546, -49.5659)
  line L349 (69.0546, -49.5659) -> (69.0594, -49.646)
  line L350 (69.0594, -49.646) -> (69.0659, -49.7253)
  line L351 (69.0659, -49.7253) -> (69.0745, -49.8038)
  line L352 (69.0745, -49.8038) -> (69.085, -49.8814)
  line L353 (69.085, -49.8814) -> (69.0978, -49.958)
  line L354 (69.0978, -49.958) -> (69.113, -50.0336)
  line L355 (69.113, -50.0336) -> (69.1309, -50.1079)
  line L356 (69.1309, -50.1079) -> (69.1521, -50.1807)
  line L357 (69.1521, -50.1807) -> (69.1783, -50.2512)
  line L358 (69.1783, -50.2512) -> (69.3538, -50.623)
  line L359 (69.3538, -50.623) -> (69.1611, -50.7169)
  line L360 (69.1611, -50.7169) -> (68.9708, -50.8156)
  line L361 (68.9708, -50.8156) -> (68.783, -50.9189)
  line L362 (68.783, -50.9189) -> (68.5979, -51.027)
  line L363 (68.5979, -51.027) -> (68.3863, -50.6746)
  line L364 (68.3863, -50.6746) -> (68.3422, -50.6137)
  line L365 (68.3422, -50.6137) -> (68.2935, -50.5556)
  line L366 (68.2935, -50.5556) -> (68.2416, -50.4994)
  line L367 (68.2416, -50.4994) -> (68.1872, -50.4448)
  line L368 (68.1872, -50.4448) -> (68.1306, -50.3915)
  line L369 (68.1306, -50.3915) -> (68.0719, -50.3396)
  line L370 (68.0719, -50.3396) -> (68.0114, -50.2889)
  line L371 (68.0114, -50.2889) -> (67.9491, -50.2394)
  line L372 (67.9491, -50.2394) -> (67.8852, -50.191)
  line L373 (67.8852, -50.191) -> (67.8196, -50.1437)
  line L374 (67.8196, -50.1437) -> (67.7526, -50.0975)
  line L375 (67.7526, -50.0975) -> (67.6841, -50.0523)
  line L376 (67.6841, -50.0523) -> (67.5733, -50.1242)
  line L377 (67.5733, -50.1242) -> (67.4635, -50.1976)
  line L378 (67.4635, -50.1976) -> (67.3547, -50.2724)
  line L379 (67.3547, -50.2724) -> (67.3702, -50.353)
  line L380 (67.3702, -50.353) -> (67.3872, -50.4326)
  line L381 (67.3872, -50.4326) -> (67.4058, -50.5113)
  line L382 (67.4058, -50.5113) -> (67.4261, -50.5889)
  line L383 (67.4261, -50.5889) -> (67.448, -50.6654)
  line L384 (67.448, -50.6654) -> (67.4717, -50.7407)
  line L385 (67.4717, -50.7407) -> (67.4972, -50.8148)
  line L386 (67.4972, -50.8148) -> (67.5247, -50.8874)
  line L387 (67.5247, -50.8874) -> (67.5543, -50.9586)
  line L388 (67.5543, -50.9586) -> (67.5864, -51.028)
  line L389 (67.5864, -51.028) -> (67.6214, -51.0953)
  line L390 (67.6214, -51.0953) -> (67.6608, -51.1593)
  line L391 (67.6608, -51.1593) -> (67.9054, -51.4897)
  line L392 (67.9054, -51.4897) -> (67.7348, -51.6194)
  line L393 (67.7348, -51.6194) -> (67.5674, -51.7533)
  line L394 (67.5674, -51.7533) -> (67.4034, -51.8913)
  line L395 (67.4034, -51.8913) -> (67.2429, -52.0334)
  line L396 (67.2429, -52.0334) -> (66.9666, -51.729)
  line L397 (66.9666, -51.729) -> (66.9115, -51.6779)
  line L398 (66.9115, -51.6779) -> (66.8524, -51.6304)
  line L399 (66.8524, -51.6304) -> (66.7905, -51.5854)
  line L400 (66.7905, -51.5854) -> (66.7265, -51.5425)
  line L401 (66.7265, -51.5425) -> (66.6606, -51.5013)
  line L402 (66.6606, -51.5013) -> (66.593, -51.4619)
  line L403 (66.593, -51.4619) -> (66.5237, -51.4239)
  line L404 (66.5237, -51.4239) -> (66.4529, -51.3875)
  line L405 (66.4529, -51.3875) -> (66.3808, -51.3525)
  line L406 (66.3808, -51.3525) -> (66.3073, -51.3189)
  line L407 (66.3073, -51.3189) -> (66.2325, -51.2867)
  line L408 (66.2325, -51.2867) -> (66.1565, -51.2557)
  line L409 (66.1565, -51.2557) -> (66.0619, -51.3479)
  line L410 (66.0619, -51.3479) -> (65.9685, -51.4412)
  line L411 (65.9685, -51.4412) -> (65.8764, -51.5359)
  line L412 (65.8764, -51.5359) -> (65.9073, -51.6119)
  line L413 (65.9073, -51.6119) -> (65.9395, -51.6867)
  line L414 (65.9395, -51.6867) -> (65.9731, -51.7602)
  line L415 (65.9731, -51.7602) -> (66.0081, -51.8323)
  line L416 (66.0081, -51.8323) -> (66.0446, -51.9031)
  line L417 (66.0446, -51.9031) -> (66.0825, -51.9723)
  line L418 (66.0825, -51.9723) -> (66.122, -52.04)
  line L419 (66.122, -52.04) -> (66.1631, -52.1059)
  line L420 (66.1631, -52.1059) -> (66.2061, -52.1699)
  line L421 (66.2061, -52.1699) -> (66.2511, -52.2317)
  line L422 (66.2511, -52.2317) -> (66.2985, -52.2909)
  line L423 (66.2985, -52.2909) -> (66.3496, -52.346)
  line L424 (66.3496, -52.346) -> (66.654, -52.6223)
  line L425 (66.654, -52.6223) -> (66.5119, -52.7828)
  line L426 (66.5119, -52.7828) -> (66.3739, -52.9468)
  line L427 (66.3739, -52.9468) -> (66.24, -53.1141)
  line L428 (66.24, -53.1141) -> (66.1103, -53.2848)
  line L429 (66.1103, -53.2848) -> (65.78, -53.0402)
  line L430 (65.78, -53.0402) -> (65.7159, -53.0008)
  line L431 (65.7159, -53.0008) -> (65.6486, -52.9658)
  line L432 (65.6486, -52.9658) -> (65.5792, -52.9337)
  line L433 (65.5792, -52.9337) -> (65.5081, -52.9041)
  line L434 (65.5081, -52.9041) -> (65.4354, -52.8766)
  line L435 (65.4354, -52.8766) -> (65.3613, -52.851)
  line L436 (65.3613, -52.851) -> (65.286, -52.8274)
  line L437 (65.286, -52.8274) -> (65.2095, -52.8055)
  line L438 (65.2095, -52.8055) -> (65.1319, -52.7852)
  line L439 (65.1319, -52.7852) -> (65.0533, -52.7666)
  line L440 (65.0533, -52.7666) -> (64.9736, -52.7495)
  line L441 (64.9736, -52.7495) -> (64.893, -52.734)
  line L442 (64.893, -52.734) -> (64.8182, -52.8429)
  line L443 (64.8182, -52.8429) -> (64.7448, -52.9527)
  line L444 (64.7448, -52.9527) -> (64.6729, -53.0634)
  line L445 (64.6729, -53.0634) -> (64.7181, -53.132)
  line L446 (64.7181, -53.132) -> (64.7643, -53.199)
  line L447 (64.7643, -53.199) -> (64.8116, -53.2646)
  line L448 (64.8116, -53.2646) -> (64.86, -53.3285)
  line L449 (64.86, -53.3285) -> (64.9096, -53.3908)
  line L450 (64.9096, -53.3908) -> (64.9602, -53.4513)
  line L451 (64.9602, -53.4513) -> (65.0122, -53.51)
  line L452 (65.0122, -53.51) -> (65.0654, -53.5666)
  line L453 (65.0654, -53.5666) -> (65.12, -53.621)
  line L454 (65.12, -53.621) -> (65.1762, -53.6728)
  line L455 (65.1762, -53.6728) -> (65.2343, -53.7216)
  line L456 (65.2343, -53.7216) -> (65.2952, -53.7657)
  line L457 (65.2952, -53.7657) -> (65.6476, -53.9773)
  line L458 (65.6476, -53.9773) -> (65.5396, -54.1624)
  line L459 (65.5396, -54.1624) -> (65.4362, -54.3502)
  line L460 (65.4362, -54.3502) -> (65.3375, -54.5405)
  line L461 (65.3375, -54.5405) -> (65.2436, -54.7331)
  line L462 (65.2436, -54.7331) -> (64.8719, -54.5577)
  line L463 (64.8719, -54.5577) -> (64.8014, -54.5315)
  line L464 (64.8014, -54.5315) -> (64.7286, -54.5103)
  line L465 (64.7286, -54.5103) -> (64.6542, -54.4924)
  line L466 (64.6542, -54.4924) -> (64.5787, -54.4772)
  line L467 (64.5787, -54.4772) -> (64.502, -54.4644)
  line L468 (64.502, -54.4644) -> (64.4244, -54.4538)
  line L469 (64.4244, -54.4538) -> (64.3459, -54.4453)
  line L470 (64.3459, -54.4453) -> (64.2666, -54.4387)
  line L471 (64.2666, -54.4387) -> (64.1865, -54.434)
  line L472 (64.1865, -54.434) -> (64.1058, -54.4311)
  line L473 (64.1058, -54.4311) -> (64.0243, -54.4299)
  line L474 (64.0243, -54.4299) -> (63.9423, -54.4304)
  line L475 (63.9423, -54.4304) -> (63.8901, -54.5518)
  line L476 (63.8901, -54.5518) -> (63.8396, -54.6738)
  line L477 (63.8396, -54.6738) -> (63.7907, -54.7964)
  line L478 (63.7907, -54.7964) -> (63.8483, -54.8548)
  line L479 (63.8483, -54.8548) -> (63.9067, -54.9116)
  line L480 (63.9067, -54.9116) -> (63.9659, -54.9666)
  line L481 (63.9659, -54.9666) -> (64.0259, -55.0199)
  line L482 (64.0259, -55.0199) -> (64.0866, -55.0713)
  line L483 (64.0866, -55.0713) -> (64.1481, -55.1208)
  line L484 (64.1481, -55.1208) -> (64.2105, -55.1682)
  line L485 (64.2105, -55.1682) -> (64.2737, -55.2134)
  line L486 (64.2737, -55.2134) -> (64.3379, -55.2561)
  line L487 (64.3379, -55.2561) -> (64.4031, -55.2959)
  line L488 (64.4031, -55.2959) -> (64.4696, -55.3324)
  line L489 (64.4696, -55.3324) -> (64.538, -55.3638)
  line L490 (64.538, -55.3638) -> (64.9249, -55.5026)
  line L491 (64.9249, -55.5026) -> (64.855, -55.7052)
  line L492 (64.855, -55.7052) -> (64.7903, -55.9095)
  line L493 (64.7903, -55.9095) -> (64.7306, -56.1154)
  line L494 (64.7306, -56.1154) -> (64.6761, -56.3227)
  line L495 (64.6761, -56.3227) -> (64.2773, -56.2231)
  line L496 (64.2773, -56.2231) -> (64.203, -56.2113)
  line L497 (64.203, -56.2113) -> (64.1275, -56.2047)
  line L498 (64.1275, -56.2047) -> (64.0511, -56.2016)
  line L499 (64.0511, -56.2016) -> (63.974, -56.2014)
  line L500 (63.974, -56.2014) -> (63.8963, -56.2038)
  line L501 (63.8963, -56.2038) -> (63.8181, -56.2086)
  line L502 (63.8181, -56.2086) -> (63.7395, -56.2156)
  line L503 (63.7395, -56.2156) -> (63.6604, -56.2246)
  line L504 (63.6604, -56.2246) -> (63.581, -56.2356)
  line L505 (63.581, -56.2356) -> (63.5012, -56.2485)
  line L506 (63.5012, -56.2485) -> (63.4211, -56.2632)